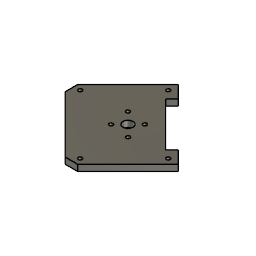
固定具 v3 (Autodesk Fusion 360 design; units mm, degrees)
Autodesk Fusion 360 part; units mm, degrees
note: some values were not read from the file. Set by a fixed rule: which sketch regions a step uses.
sketch "スケッチ1" plane through (0, 0, 0) normal (0, 0, 1) x (1, 0, 0)
  line L0 (55, 0) -> (45, 0)
  line L1 (45, 0) -> (0, 45)
  line L2 (0, 45) -> (0, 55)
  line L3 (0, 55) -> (40, 95)
  line L4 (40, 95) -> (95, 40)
  line L5 (95, 40) -> (55, 0)
  constraint horizontal L0
  constraint perpendicular L0 L2
  constraint perpendicular L3 L4
extrude "押し出し1" add sketch "スケッチ1" along normal blind 5
sketch "スケッチ2" plane through (0, 0, 5) normal (0, 0, 1) x (-1, 0, 0)
  line L0 (-95, -40) -> (-40, -95)
  line L1 (-40, -95) -> (0, -55)
  line L2 (0, -55) -> (0, -45)
  line L3 (0, -45) -> (-45, 0)
  line L4 (-45, 0) -> (-55, 0)
  line L5 (-55, 0) -> (-95, -40)
  line L6 (-55, -10) -> (-80, -35)
  line L7 (-80, -45) -> (-45, -80)
  line L8 (-35, -80) -> (-10, -55)
  line L9 (-10, -55) -> (-55, -10)
  line L10 (-35, -80) -> (-45, -80)
  line L11 (-80, -45) -> (-80, -35)
  line L12 (-62.5, -62.5) -> (-32.5, -32.5)
  circle A0 centre (-47.5, -47.5) radius 21.225
  circle A1 centre (-40.7825, -40.7825) radius 1.5
  circle A2 centre (-56.3388, -38.6612) radius 1.5
  circle A3 centre (-54.2175, -54.2175) radius 1.5
  circle A4 centre (-38.6612, -56.3388) radius 1.5
  line L13 (-38.6612, -56.3388) -> (-56.3388, -38.6612)
  circle A5 centre (-47.5, -47.5) radius 4
  point P0 (-47.5, -47.5)
  dimension "d4" = 3
  dimension "d11" = 19
  dimension "d12" = 12.5
  dimension "d13" = 12.5
  dimension "d14" = 3
  dimension "d15" = 3
  dimension "d16" = 3
  dimension "d17" = 8
  constraint perpendicular L0 L6
  constraint perpendicular L6 L7
  constraint perpendicular L7 L8
  constraint perpendicular L6 L9
  constraint horizontal L10
  constraint perpendicular L10 L11
  constraint midpoint L7 L12.start
  constraint midpoint L9 L12.end
  constraint perpendicular L9 L12
  constraint midpoint L12 P0
  constraint coincident L12 A1.centre
  constraint coincident A4.centre L13.start
  constraint coincident A2.centre L13.end
  constraint coincident P0 A0.centre
  measures "d4" diameter of A1
  measures "d11" distance of A1.centre A3.centre
  measures "d12" distance of P0 A4.centre
  measures "d13" distance of P0 A2.centre
  measures "d14" diameter of A4
  measures "d15" diameter of A3
  measures "d16" diameter of A2
  measures "d17" diameter of A5
sketch "スケッチ3" plane through (0, 0, 5) normal (0, 0, 1) x (-1, 0, 0)
  circle A0 centre (-5, -52) radius 1.5
  circle A1 centre (-52, -5) radius 1.5
  circle A2 centre (-40, -87) radius 1.5
  circle A3 centre (-87, -40) radius 1.5
extrude "押し出し2" cut sketch "スケッチ3" sketch "スケッチ2" against normal blind 5 of sketch 2 contours L12 A1 | L12 A1 | L12 A3 | L12 A3 | A2 | A4
sketch "スケッチ4" plane through (0, 0, 0) normal (0, 0, -1) x (1, 0, 0)
  line L0 (40, -95) -> (95, -40)
  line L1 (95, -40) -> (55, 0)
  line L2 (55, 0) -> (45, 0)
  line L3 (45, 0) -> (0, -45)
  line L4 (0, -45) -> (0, -55)
  line L5 (0, -55) -> (40, -95)
  circle A0 centre (38.6612, -56.3388) radius 1.5
  circle A1 centre (54.2175, -54.2175) radius 1.5
  circle A2 centre (87, -40) radius 1.5
  circle A3 centre (40, -87) radius 1.5
  circle A4 centre (52, -5) radius 1.5
  circle A5 centre (5, -52) radius 1.5
  circle A6 centre (40.7825, -40.7825) radius 1.5
  circle A7 centre (56.3388, -38.6612) radius 1.5
  line L6 (85, -50) -> (80, -45)
  line L7 (80, -45) -> (45, -80)
  line L8 (45, -80) -> (50, -85)
  line L9 (85, -50) -> (50, -85)
  constraint coincident L0 L6.start
  constraint perpendicular L0 L6
  constraint perpendicular L6 L7
  constraint coincident L0 L8.end
  constraint perpendicular L0 L8
extrude "押し出し3" cut sketch "スケッチ4" against normal blind 5 contours L0 L6 L7 L8 L9
extrude "押し出し4" cut sketch "スケッチ2" against normal blind 12 contours L12 L13 A5 | L12 L13 A5 | L12 L13 A5 | L12 L13 A5
